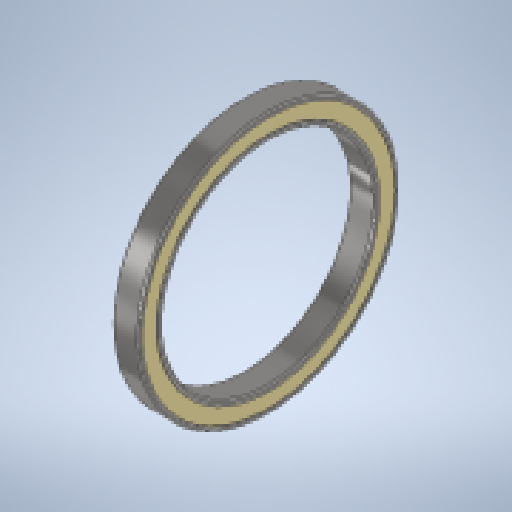
# Autodesk Inventor part: Bearing_Large
Saved by Autodesk Inventor 2024 (Build 280153000, 153)
## iProperties
Created: 2024-06-23
Part Number: Bearing_Large
Material: 一般
Document SubType Name: Modeling
Designer: tanoue_kota
Density: 6.10081 g/cm^3
Appearance: 鋼 - つや出し
Mass: 340 g
Surface Area: 192.285 cm^2
Volume: 55.7303 cm^3
Author: tanoue_kota
Autodesk Inventor part; units mm, degrees
ref_plane "YZ Plane" through (0, 0, 0) normal (1, 0, 0) x (0, 1, 0)
ref_plane "XZ Plane" through (0, 0, 0) normal (0, 1, 0) x (-1, 0, 0)
ref_plane "XY Plane" through (0, 0, 0) normal (0, 0, 1) x (1, 0, 0)
sketch "スケッチ1" plane through (0, 0, 0) normal (1, 0, 0) x (0, 1, 0)
  circle A0 centre (0, 0) radius 65
  circle A1 centre (0, 0) radius 52.5
  dimension "d0" = 130
  dimension "d1" = 105
  constraints: 2 centre point, 2 coincident
  measures "d0" diameter of A0
  measures "d1" diameter of A1
extrude "押し出し1" add sketch "スケッチ1" along normal blind 13
fillet "フィレット1" radius 1 4 edges at (13, -65, 0) (0, -65, 0) (13, -52.5, 0) (0, -52.5, 0)
sketch "スケッチ2" plane through (13, 0, 0) normal (1, 0, 0) x (0, 0, -1)
  circle A0 centre (0, 0) radius 55.1
  circle A1 centre (0, 0) radius 52.5 projected
  circle A2 centre (0, 0) radius 62.7
  circle A3 centre (0, 0) radius 65 projected
  dimension "d5" = 2.6
  dimension "d6" = 2.3
  constraints: 2 centre point, 2 coincident
  measures "d5" radial gap between concentric circles of A1 A0
  measures "d6" radial gap between concentric circles of A3 A2
extrude "押し出し2" cut sketch "スケッチ2" against normal blind 0.7 contours A2
sketch "スケッチ3" plane through (0, 0, 0) normal (-1, 0, 0) x (0, 0, 1)
  circle A0 centre (0, 0) radius 55.1
  circle A1 centre (0, 0) radius 62.7
  constraints: 2 centre point, 2 coincident
extrude "押し出し3" cut sketch "スケッチ3" against normal blind 0.7
